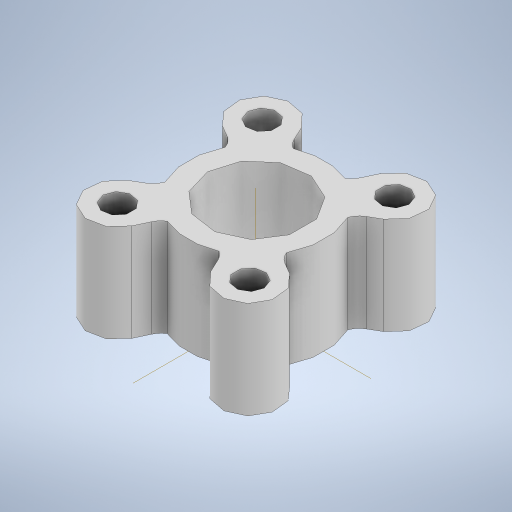
# Autodesk Inventor part: крепление подшипника_1
Saved by Autodesk Inventor 2024.2 (Build 282272000, 272)
## iProperties
Created: 2025-11-25
Part Number: крепление подшипника_1
Material: Типовые
Document SubType Name: Modeling
Designer: Zakhar
Density: 1 g/cm^3
Appearance: По умолчанию
Author: Zakhar
Autodesk Inventor part; units mm, degrees
ref_plane "YZ Plane" through (0, 0, 0) normal (1, 0, 0) x (0, 1, 0)
ref_plane "XZ Plane" through (0, 0, 0) normal (0, 1, 0) x (-1, 0, 0)
ref_plane "XY Plane" through (0, 0, 0) normal (0, 0, 1) x (1, 0, 0)
sketch "Эскиз1" plane through (0, 0, 0) normal (0, 1, 0) x (-1, 0, 0)
  circle A0 centre (-0.0254, 0) radius 7
  circle A1 centre (-7.0254, 6.889) radius 1.5
  circle A2 centre (6.7752, 7.433) radius 1.5
  circle A3 centre (6.9746, -7.0215) radius 1.5
  circle A4 centre (-7.0254, -7.0215) radius 1.5
  circle A5 centre (-0.0254, 0) radius 5
  line L0 (0, 0) -> (0, 8.1981) construction
  line L1 (-0.0254, 0) -> (8.1589, 0) construction
  circle A6 centre (6.7752, 7.433) radius 3
  line L2 (4.0592, 8.7071) -> (3.4025, 7.3072)
  line L3 (8.2851, 4.8407) -> (7.1407, 4.1741)
  line L4 (0.7424, 6.346) -> (0.4551, 6.4808)
  arc A7 (0.7424, 6.346) -> (3.4025, 7.3072) centre (1.5918, 8.1566) ccw
  line L5 (5.7914, 2.5169) -> (6.4192, 1.4392)
  arc A8 (7.1407, 4.1741) -> (6.4192, 1.4392) centre (8.1474, 2.4459) ccw
  point P0 (-10.336, -7.0215)
  point P1 (-9.1433, 6.8618)
  point P2 (6.9746, 10.1261)
  point P3 (2.6587, 6.4649)
  point P4 (6.2546, 3.0921)
  dimension "d0" = 14
  dimension "d1" = 3
  dimension "d2" = 3
  dimension "d3" = 3
  dimension "d4" = 3
  dimension "d5" = 10
  dimension "d6" = 6
  dimension "d7" = 2
  dimension "d8" = 2
  constraints: 12 end point, 9 centre point, 6 point on circle, 6 tangent, 3 point on line, 2 coincident, 2 perpendicular, 1 horizontal, 1 vertical
  measures "d0" diameter of A0
  measures "d1" diameter of A1
  measures "d2" diameter of A2
  measures "d3" diameter of A3
  measures "d4" diameter of A4
  measures "d5" diameter of A5
  measures "d6" diameter of A6
  measures "d7" radius of A7
  measures "d8" radius of A8
extrude "Выдавливание1" add sketch "Эскиз1" along normal blind 10 contours A0
extrude "Выдавливание2" add sketch "Эскиз1" along normal blind 10 contours A0 A7 L2 A6 L3 A8 | A6
mirror "Зеркальное отражение1" about plane through (0, 0, 0) normal (1, 0, 0) of "Выдавливание2"
mirror "Зеркальное отражение2" about plane through (0, 0, 0) normal (0, 0, 1) of "Выдавливание2", "Зеркальное отражение1"
